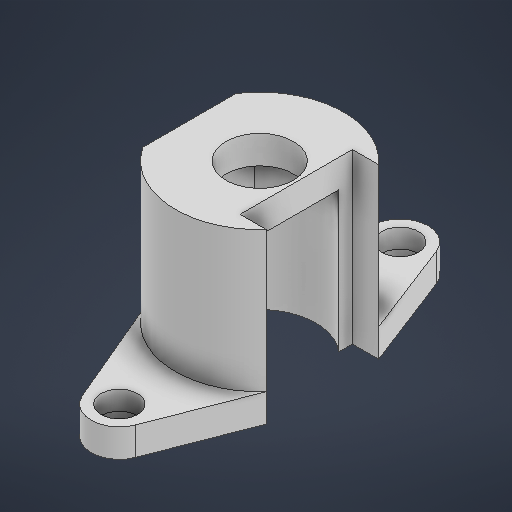
# Autodesk Inventor part: motor mount
Saved by Autodesk Inventor 2025.2 (Build 292293000, 293)
## iProperties
Created: 2025-05-21
Part Number: motor mount
Material: Generic
Document SubType Name: Modeling
Designer: klawy
Density: 1 g/cm^3
Appearance: Default
Author: klawy
Autodesk Inventor part; units mm, degrees
ref_plane "YZ Plane" through (0, 0, 0) normal (1, 0, 0) x (0, 1, 0)
ref_plane "XZ Plane" through (0, 0, 0) normal (0, 1, 0) x (-1, 0, 0)
ref_plane "XY Plane" through (0, 0, 0) normal (0, 0, 1) x (1, 0, 0)
sketch "Sketch1" plane through (0, 0, 0) normal (0, 1, 0) x (-1, 0, 0)
  line L0 (-7.5, 6.6144) -> (7.5, 6.6144) construction
  line L1 (7.5, 6.6144) -> (7.5, -6.6144)
  line L2 (7.5, -6.6144) -> (-7.5, -6.6144) construction
  line L3 (-7.5, -6.6144) -> (-7.5, 6.6144)
  line L4 (-7.5, 6.6144) -> (7.5, -6.6144) construction
  line L5 (7.5, 6.6144) -> (-7.5, -6.6144) construction
  arc A0 (7.5, 6.6144) -> (-7.5, 6.6144) centre (0, 0) ccw
  arc A1 (-7.5, -6.6144) -> (7.5, -6.6144) centre (0, 0) ccw
  line L6 (-12.5, 8.2916) -> (-12.5, -8.2916)
  arc A2 (-12.5, -8.2916) -> (12.5, -8.2916) centre (0, 0) ccw
  line L7 (12.5, -8.2916) -> (12.5, 8.2916)
  arc A3 (12.5, 8.2916) -> (-12.5, 8.2916) centre (0, 0) ccw
  dimension "d1" = 15
  dimension "d2" = 10
  dimension "d3" = 5
  constraints: 16 end point, 8 point on circle, 4 centre point, 3 parallel, 2 midpoint, 1 coincident, 1 horizontal, 1 perpendicular, 3 other
  measures "d1" distance of L0.start L0.end
  measures "d2" radius of A0
  measures "d3" radial gap between concentric circles of A0 A3
extrude "Extrusion1" add sketch "Sketch1" along normal blind 25
sketch "Sketch2" plane through (0, 25, 0) normal (0, 1, 0) x (1, 0, 0)
  arc A0 (12.5, 8.2916) -> (-12.5, 8.2916) centre (0, 0) ccw projected
  line L0 (-12.5, 8.2916) -> (-12.5, -8.2916) projected
  arc A1 (-12.5, -8.2916) -> (12.5, -8.2916) centre (0, 0) ccw projected
  line L1 (12.5, -8.2916) -> (12.5, 8.2916) projected
  line L2 (7.5, 6.6144) -> (7.5, -6.6144) projected
  arc A2 (-7.5, -6.6144) -> (7.5, -6.6144) centre (0, 0) ccw projected
  line L3 (-7.5, -6.6144) -> (-7.5, 6.6144) projected
  arc A3 (7.5, 6.6144) -> (-7.5, 6.6144) centre (0, 0) ccw projected
  circle A4 centre (0, 0) radius 6
  dimension "d6" = 12
  constraints: 1 centre point, 1 coincident
  measures "d6" diameter of A4
extrude "Extrusion2" add sketch "Sketch2" along normal blind 5 contours L1 A1 L0 A0 | L2 A2 L3 A3
sketch "Sketch3" plane through (12.5, 0, 8.2916) normal (1, 0, 0) x (0, 0, -1)
  line L0 (18.2916, 18) -> (-1.7084, 18)
  line L1 (-1.7084, 18) -> (-1.7084, 30)
  line L2 (-1.7084, 30) -> (18.2916, 30)
  line L3 (18.2916, 30) -> (18.2916, 18)
  line L4 (0, 30) -> (16.5831, 30) projected
  point P0 (8.2916, 0)
  point P1 (8.2916, 30)
  dimension "d9" = 12
  dimension "d10" = 20
  constraints: 8 end point, 2 midpoint, 2 parallel, 1 horizontal, 1 perpendicular
  measures "d9" distance of L2.end L0.start
  measures "d10" distance of L1.end L2.end
extrude "Extrusion3" cut sketch "Sketch3" against normal blind 6
sketch "Sketch4" plane through (12.5, 18, 8.2916) normal (0, 1, 0) x (1, 0, 0)
  arc A0 (-1.3197, -1.7084) -> (0, 0) centre (-12.5, 8.2916) ccw projected
  line L0 (0, 16.5831) -> (0, 0) projected
  arc A1 (0, 16.5831) -> (-1.3197, 18.2916) centre (-12.5, 8.2916) ccw projected
  line L1 (-1.3197, 18.2916) -> (-6, 18.2916) projected
  line L2 (-6, 18.2916) -> (-6, 15.8909) projected
  arc A2 (-5, 14.9059) -> (-6, 15.8909) centre (-12.5, 8.2916) ccw projected
  line L3 (-5, 1.6772) -> (-5, 14.9059) projected
  arc A3 (-6, 0.6922) -> (-5, 1.6772) centre (-12.5, 8.2916) ccw projected
  line L4 (-6, 0.6922) -> (-6, -1.7084) projected
  line L5 (-1.3197, -1.7084) -> (-6, -1.7084) projected
  point P0 (-12.5, 8.2916)
extrude "Extrusion4" cut sketch "Sketch4" against normal through all
sketch "Sketch5" plane through (0, 0, 0) normal (0, -1, 0) x (1, 0, 0)
  line L0 (6.5, -10) -> (6.5, -7.5993) projected
  arc A0 (-7.5, -6.6144) -> (6.5, -7.5993) centre (0, 0) ccw projected
  line L1 (-7.5, 6.6144) -> (-7.5, -6.6144) projected
  arc A1 (6.5, 7.5993) -> (-7.5, 6.6144) centre (0, 0) ccw projected
  line L2 (6.5, 7.5993) -> (6.5, 10) projected
  line L3 (6.5, 10) -> (11.1803, 10) projected
  arc A2 (11.1803, 10) -> (-12.5, 8.2916) centre (0, 0) ccw projected
  line L4 (-12.5, -8.2916) -> (-12.5, 8.2916) projected
  arc A3 (-12.5, -8.2916) -> (11.1803, -10) centre (0, 0) ccw projected
  line L5 (11.1803, -10) -> (6.5, -10) projected
  line L6 (0, 25) -> (0, -25)
  circle A4 centre (0, 25) radius 5
  circle A5 centre (0, -25) radius 5
  line L7 (4.6617, 26.8079) -> (11.1803, 10)
  line L8 (11.1803, -10) -> (4.6617, -26.8079)
  line L9 (-4.6047, -26.9486) -> (-12.5, -8.2916)
  line L10 (-12.5, 8.2916) -> (-4.6047, 26.9486)
  dimension "d15" = 50
  dimension "d16" = 10
  dimension "d17" = 10
  constraints: 10 end point, 4 point on circle, 4 tangent, 3 coincident, 2 centre point, 1 midpoint, 1 vertical
  measures "d15" distance of L6.start L6.end
  measures "d16" diameter of A4
  measures "d17" diameter of A5
extrude "Extrusion5" add sketch "Sketch5" against normal blind 5 contours L8 A5 L6 A3 | L6 A5 L9 A3 | A5 | L6 A4 L7 A2 | A2 L10 A4 L6 | A4
sketch "Sketch6" plane through (0, 5, 0) normal (0, 1, 0) x (1, 0, 0)
  line L0 (-12.5, -8.2916) -> (-4.6047, -26.9486) projected
  arc A0 (-4.6047, -26.9486) -> (4.6617, -26.8079) centre (0, -25) ccw projected
  line L1 (4.6617, -26.8079) -> (11.1803, -10) projected
  arc A1 (-12.5, -8.2916) -> (11.1803, -10) centre (0, 0) ccw projected
  arc A2 (11.1803, 10) -> (-12.5, 8.2916) centre (0, 0) ccw projected
  line L2 (11.1803, 10) -> (4.6617, 26.8079) projected
  arc A3 (4.6617, 26.8079) -> (-4.6047, 26.9486) centre (0, 25) ccw projected
  line L3 (-4.6047, 26.9486) -> (-12.5, 8.2916) projected
  constraints: 2 coincident
hole "Hole1" at (0, 5, 25) at (0, 5, -25) direction (0, -1, 0) diameter 3.4 end through all counterbore diameter 6.5 counterbore depth 3.4 clearance for "Socket Head Cap Screw ISO 4762" size "M3" standard "ISO"
body "Solid1"
